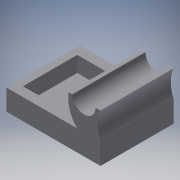
# Autodesk Inventor part: Y_Fixture_Motor
Saved by Autodesk Inventor 2019.3 (Build 233278000, 278)
## iProperties
Created: 2020-09-01
Part Number: Y_Fixture_Motor
Material: Generisch
Document SubType Name: Modeling
Designer: Nicolas Frick
Density: 1 g/cm^3
Appearance: Vorgabe
Author: Nicolas Frick
Autodesk Inventor part; units mm, degrees
ref_plane "YZ Plane" through (0, 0, 0) normal (1, 0, 0) x (0, 1, 0)
ref_plane "XZ Plane" through (0, 0, 0) normal (0, 1, 0) x (-1, 0, 0)
ref_plane "XY Plane" through (0, 0, 0) normal (0, 0, 1) x (1, 0, 0)
sketch "Skizze8" plane through (0, 0, 0) normal (0, 0, 1) x (1, 0, 0)
  line L0 (1091.5011, -38.4824) -> (-8.4811, -32.2289) construction
  circle A0 centre (10.7, 0) radius 11 construction
  line L1 (942.3125, 104.6681) -> (32.3272, 109.8414) construction
  line L2 (942.3125, 104.6681) -> (941.5223, -34.3297) construction
  line L3 (31.537, -29.1563) -> (941.5223, -34.3297) construction
  line L4 (32.3272, 109.8414) -> (31.537, -29.1563) construction
  circle A1 centre (10.7, 0) radius 11.125
  line L5 (1091.4244, -51.9822) -> (-8.5578, -45.7286) construction
  line L6 (26.537, -45.9282) -> (-63.463, -45.9282)
  line L7 (-63.463, -45.9282) -> (-63.463, -25.9282)
  line L8 (-3.9718, 0) -> (26.537, 0)
  line L9 (26.537, -25.2811) -> (26.537, -45.9282)
  line L10 (-0.425, 0) -> (-3.9718, 0)
  line L11 (-63.463, -45.9282) -> (-63.463, -25.9282)
  line L12 (-63.463, -25.9282) -> (1.4698, -25.9282)
  arc A2 (26.537, 0) -> (26.537, -25.2811) centre (55.0132, -12.6406) ccw
  line L13 (-63.463, -25.9282) -> (4.0847, -25.9282)
  arc A3 (-3.9718, 0) -> (4.0847, -25.9282) centre (26.3099, -4.8066) ccw
  point P0 (0, 0)
  dimension "d72" = 20
  constraints: 18 end point, 4 point on circle, 3 horizontal, 2 centre point, 2 parallel, 2 point on line, 1 coincident, 1 horizontal alignment, 1 perpendicular, 5 other
  measures "d72" distance of L7.end L6.end
extrude "Extrusion9" add sketch "Skizze8" along normal blind 70 contours L8 A2 L9 L6 L7 L12 L13 A3 A1 | A1 L8 picked at (11.147, -3.6813)
sketch "Skizze9" plane through (-63.463, -25.9282, 0) normal (0, 1, 0) x (1, 0, 0)
  circle A0 centre (28, -35) radius 5 construction
  circle A1 centre (12.5, -50.5) radius 3 construction
  circle A2 centre (43.5, -50.5) radius 3 construction
  circle A3 centre (12.5, -19.5) radius 3 construction
  circle A4 centre (43.5, -19.5) radius 3 construction
  arc A5 (36, -10.5) -> (35.5, -10) centre (35.5, -10.5) ccw construction
  line L0 (35.5, -10) -> (20.5, -10) construction
  arc A6 (20.5, -10) -> (20, -10.5) centre (20.5, -10.5) ccw construction
  line L1 (20, -10.5) -> (20, -14) construction
  line L2 (20, -14) -> (13, -14) construction
  line L3 (13, -14) -> (7, -20) construction
  line L4 (7, -20) -> (7, -50) construction
  line L5 (7, -50) -> (13, -56) construction
  line L6 (13, -56) -> (43, -56) construction
  line L7 (43, -56) -> (49, -50) construction
  line L8 (49, -50) -> (49, -20) construction
  line L9 (49, -20) -> (43, -14) construction
  line L10 (43, -14) -> (36, -14) construction
  line L11 (36, -14) -> (36, -10.5) construction
  line L12 (49.15, -61) -> (6.85, -61)
  line L13 (6.85, -61) -> (6.85, -9)
  line L14 (6.85, -9) -> (49.15, -9)
  line L15 (49.15, -9) -> (49.15, -61)
  line L16 (49.15, -61) -> (6.85, -9) construction
  line L17 (6.85, -61) -> (49.15, -9) construction
  point P0 (63.463, 0)
  dimension "d75" = 42.3
  dimension "d76" = 52
  constraints: 12 end point, 2 midpoint, 2 parallel, 1 horizontal, 1 perpendicular
  measures "d75" distance of L13.end L14.end
  measures "d76" distance of L12.end L13.end
extrude "Extrusion10" cut sketch "Skizze9" against normal blind 15
sketch "Skizze11" plane through (0, 0, 0) normal (0, 0, -1) x (-1, 0, 0)
  circle A0 centre (-10.7, 0) radius 11 construction
  arc A1 (-21.825, 0) -> (0.425, 0) centre (-10.7, 0) ccw
  line L0 (0, 0) -> (-21.825, 0)
  line L1 (-26.537, 0) -> (3.9718, 0) projected
  dimension "d79" = 22.25
  constraints: 2 end point, 2 point on circle, 2 point on line, 1 centre point, 1 coincident
  measures "d79" diameter of A1
extrude "Extrusion11" cut sketch "Skizze11" against normal through all
